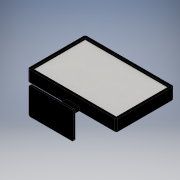
# Autodesk Inventor part: Ecran
Saved by Autodesk Inventor 2016 SP1 (Build 200210100, 210)
## iProperties
Created: 2016-10-04
Part Number: Ecran
Material: Générique
Document SubType Name: Modeling
Designer: dimercur
Density: 1 g/cm^3
Appearance: Noir
Author: dimercur
Autodesk Inventor part; units mm, degrees
ref_plane "YZ Plane" through (0, 0, 0) normal (1, 0, 0) x (0, 1, 0)
ref_plane "XZ Plane" through (0, 0, 0) normal (0, 1, 0) x (-1, 0, 0)
ref_plane "XY Plane" through (0, 0, 0) normal (0, 0, 1) x (1, 0, 0)
sketch "Esquisse1" plane through (0, 0, 0) normal (0, 0, 1) x (1, 0, 0)
  line L0 (-242.3239, 202.8486) -> (312.6761, 202.8486)
  line L1 (312.6761, 202.8486) -> (312.6761, -157.1514)
  line L2 (312.6761, -157.1514) -> (-242.3239, -157.1514)
  line L3 (-242.3239, -157.1514) -> (-242.3239, 202.8486)
  point P0 (0, 0)
  dimension "d0" = 555
  dimension "d1" = 360
  constraints: 8 end point, 2 parallel, 1 horizontal, 1 perpendicular
  measures "d0" distance of L0.start L0.end
  measures "d1" distance of L2.end L0.start
extrude "Extrusion1" add sketch "Esquisse1" along normal blind 70
fillet "Congé1" radius 10 4 edges at (-242.3239, 202.8486, 35) (-242.3239, -157.1514, 35) (312.6761, -157.1514, 35) (312.6761, 202.8486, 35)
sketch "Esquisse2" plane through (0, 0, 70) normal (0, 0, 1) x (1, 0, 0)
  line L0 (-227.3239, 187.8486) -> (297.6761, 187.8486)
  line L1 (297.6761, 187.8486) -> (297.6761, -142.1514)
  line L2 (297.6761, -142.1514) -> (-227.3239, -142.1514)
  line L3 (-227.3239, -142.1514) -> (-227.3239, 187.8486)
  line L4 (302.6761, 202.8486) -> (-232.3239, 202.8486) projected
  line L5 (-232.3239, -157.1514) -> (302.6761, -157.1514) projected
  line L6 (-242.3239, 192.8486) -> (-242.3239, -147.1514) projected
  line L7 (312.6761, -147.1514) -> (312.6761, 192.8486) projected
  point P0 (0, 0)
  dimension "d5" = 15
  dimension "d6" = 15
  dimension "d7" = 15
  dimension "d8" = 15
  constraints: 8 end point, 2 parallel, 1 horizontal, 1 perpendicular
  measures "d5" distance between parallel lines of L0 L4
  measures "d6" distance between parallel lines of L5 L2
  measures "d7" distance between parallel lines of L3 L6
  measures "d8" distance between parallel lines of L7 L1
extrude "Extrusion2" cut sketch "Esquisse2" against normal blind 10
sketch "Esquisse3" plane through (-232.3239, -157.1514, 0) normal (0, -1, 0) x (1, 0, 0)
  line L0 (232.3239, 0) -> (312.3239, 0)
  line L1 (312.3239, 0) -> (312.3239, 25)
  line L2 (312.3239, 25) -> (232.3239, 25)
  line L3 (232.3239, 25) -> (232.3239, 0)
  dimension "d11" = 80
  dimension "d12" = 25
  constraints: 8 end point, 2 parallel, 1 horizontal, 1 perpendicular
  measures "d11" distance of L1.end L2.end
  measures "d12" distance between parallel lines of L0 L2
extrude "Extrusion3" add sketch "Esquisse3" along normal blind 120
sketch "Esquisse4" plane through (-232.3239, -277.1514, 0) normal (0, -1, 0) x (1, 0, 0)
  line L0 (132.3239, 120) -> (412.3239, 120)
  line L1 (412.3239, 120) -> (412.3239, -50)
  line L2 (412.3239, -50) -> (132.3239, -50)
  line L3 (132.3239, -50) -> (132.3239, 120)
  line L4 (232.3239, 25) -> (232.3239, 0) projected
  dimension "d15" = 170
  dimension "d16" = 280
  dimension "d17" = 50
  dimension "d18" = 100
  constraints: 8 end point, 2 parallel, 1 horizontal, 1 perpendicular
  measures "d15" distance of L2.end L0.start
  measures "d16" distance of L0.start L0.end
  measures "d17" vertical distance of L4.end L2.end
  measures "d18" distance between parallel lines of L4 L3
extrude "Extrusion4" add sketch "Esquisse4" along normal blind 15
fillet "Congé2" radius 10 4 edges at (180, -284.6514, 120) (-100, -284.6514, 120) (180, -284.6514, -50) (-100, -284.6514, -50)
fillet "Congé3" radius 5 8 edges at (177.0711, -277.1514, 117.0711) (180, -277.1514, 35) (177.0711, -277.1514, -47.0711) (40, -277.1514, -50) (-97.0711, -277.1514, -47.0711) (-100, -277.1514, 35) (-97.0711, -277.1514, 117.0711) (40, -277.1514, 120)
equation "\"d6\" = d5"
equation "\"d7\" = d5"
equation "\"d8\" = d5"
